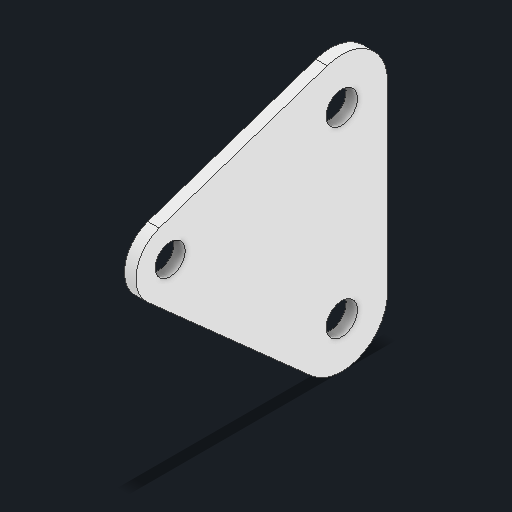
# Autodesk Inventor part: Odom Pod Gusset
Saved by Autodesk Inventor 2025.1 (Build 291241000, 241)
## iProperties
Created: 2025-01-13
Part Number: Odom Pod Gusset
Material: Acetal Resin, White
Document SubType Name: Modeling
Designer: avere
Density: 1.425 g/cm^3
Appearance: Smooth - White
Author: avere
Autodesk Inventor part; units mm, degrees
ref_plane "YZ Plane" through (0, 0, 0) normal (1, 0, 0) x (0, 1, 0)
ref_plane "XZ Plane" through (0, 0, 0) normal (0, 1, 0) x (-1, 0, 0)
ref_plane "XY Plane" through (0, 0, 0) normal (0, 0, 1) x (1, 0, 0)
sketch "Sketch1" plane through (0, 0, 0) normal (1, 0, 0) x (0, 1, 0)
  circle A0 centre (-13.9716, -13.3924) radius 2.1844
  circle A1 centre (11.4284, -13.3924) radius 2.1844
  circle A2 centre (5.0784, 10.4201) radius 2.0955
  arc A3 (11.4284, -19.7424) -> (17.4458, -11.3644) centre (11.4284, -13.3924) ccw
  arc A4 (-18.7169, -9.1728) -> (-13.9716, -19.7424) centre (-13.9716, -13.3924) ccw
  arc A5 (9.5915, 11.9411) -> (1.5194, 13.5848) centre (5.0784, 10.4201) ccw
  line L0 (17.4458, -11.3644) -> (9.5915, 11.9411)
  line L1 (1.5194, 13.5848) -> (-18.7169, -9.1728)
  line L2 (11.4284, -19.7424) -> (-13.9716, -19.7424)
  point P0 (0, 0)
  dimension "d0" = 4.191
  dimension "d1" = 12.7
  dimension "d2" = 9.525
  dimension "d3" = 12.7
  constraints: 6 centre point, 6 end point, 6 point on circle, 5 tangent, 3 coincident, 1 other
  measures "d0" diameter of A2
  measures "d1" diameter of A3
  measures "d2" diameter of A5
  measures "d3" diameter of A4
extrude "Extrusion1" add sketch "Sketch1" along normal blind 1.5875
body "Solid1"
